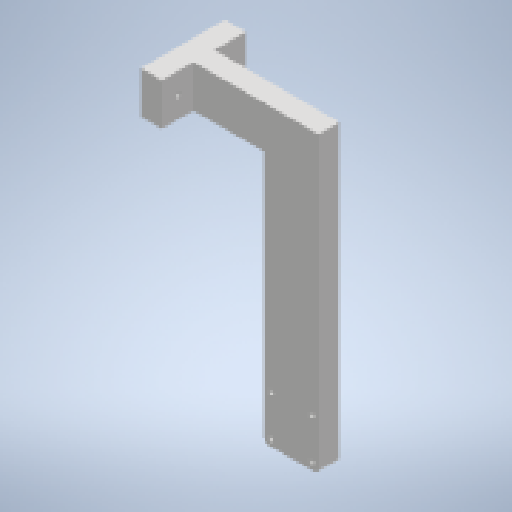
# Autodesk Inventor part: patas2
Saved by Autodesk Inventor 2023.2 (Build 272271030, 271C)
## iProperties
Created: 2023-03-05
Part Number: patas2
Material: Generic
Document SubType Name: Sheet Metal
Designer: angel
Density: 1 g/cm^3
Sheet Metal Rule: Default_mm
Appearance: Default
Author: angel
Autodesk Inventor part; units mm, degrees
ref_plane "YZ Plane" through (0, 0, 0) normal (1, 0, 0) x (0, 1, 0)
ref_plane "XZ Plane" through (0, 0, 0) normal (0, 1, 0) x (-1, 0, 0)
ref_plane "XY Plane" through (0, 0, 0) normal (0, 0, 1) x (1, 0, 0)
sketch "Sketch1" plane through (0, 0, 0) normal (0, 0, 1) x (1, 0, 0)
  line L0 (11.35, 40) -> (11.35, -15)
  line L1 (6.35, -20) -> (-48.65, -20)
  circle A0 centre (2.814466, -11.464466) radius 3
  circle A1 centre (-45.114466, -11.464466) radius 3
  circle A2 centre (-45.114466, 36.464466) radius 3
  circle A3 centre (2.814466, 36.464466) radius 3
  line L2 (-162.568945, -644.9995) -> (-162.568945, 135.0005)
  line L3 (11.35, -15) -> (11.35, 330)
  line L4 (-53.65, -15) -> (-53.65, 40)
  line L5 (-53.65, -15) -> (-53.65, 280)
  line L6 (11.35, 330) -> (-162.568945, 330)
  line L7 (-162.568945, 330) -> (-162.568945, 280)
  line L8 (-162.568945, 280) -> (-53.65, 280)
  line L9 (6.35, -20) -> (-48.65, -20)
  arc A4 (6.35, -20) -> (11.35, -15) centre (6.35, -15) ccw
  arc A5 (-53.65, -15) -> (-48.65, -20) centre (-48.65, -15) ccw
  circle A6 centre (2.814466, 36.464466) radius 3
  circle A7 centre (2.814466, -11.464466) radius 3
  circle A8 centre (-45.114466, -11.464466) radius 3
  circle A9 centre (-45.114466, 36.464466) radius 3
  point P0 (0, 0)
  dimension "d0" = 350
  dimension "d1" = 300
  dimension "d2" = 5
  measures "d0" distance from line of L3.end L1
  measures "d1" distance from line of L5.end L1
  measures "d2" radius of A4
sketch "Sketch2" plane through (-162.568945, 280, 0) normal (-1, 0, 0) x (0, 0, 1)
  line L0 (0, 0) -> (25, 0)
  line L1 (0, 50) -> (25, 50)
  line L2 (25, 0) -> (25, 50)
  line L3 (-37.5, 50) -> (62.5, 50)
  line L4 (62.5, 50) -> (62.5, 0)
  line L5 (62.5, 0) -> (-37.5, 0)
  line L6 (-37.5, 0) -> (-37.5, 50)
  circle A0 centre (42.5, 25) radius 3
  circle A1 centre (-17.5, 25) radius 3
  point P0 (0, -280)
  point P1 (12.5, 50)
  point P2 (12.5, 50)
  point P3 (62.5, 25)
  point P4 (-37.5, 25)
  dimension "d4" = 50
  dimension "d5" = 50
  dimension "d6" = 25
  dimension "d7" = 20
  dimension "d8" = 20
  dimension "d9" = 6
  measures "d4" distance from line of L4 point (12.5, 50)
  measures "d5" distance from line of L6 point (12.5, 50)
  measures "d6" distance from line of L3 point (62.5, 25)
  measures "d7" distance of A1.centre point (-37.5, 25)
  measures "d8" distance from line of L4 A0.centre
  measures "d9" diameter of A0
sketch "Sketch1 outline for Plate1" plane through (0, 0, 0) normal (0, 0, 1) x (1, 0, 0)
  arc A0 (6.35, -20) -> (11.35, -15) centre (6.35, -15) ccw
  line L0 (-48.65, -20) -> (6.35, -20)
  line L1 (11.35, -15) -> (11.35, 330)
  arc A1 (-53.65, -15) -> (-48.65, -20) centre (-48.65, -15) ccw
  line L2 (11.35, 330) -> (-162.568945, 330)
  line L3 (-53.65, 280) -> (-53.65, -15)
  line L4 (-162.568945, 330) -> (-162.568945, 280)
  line L5 (-162.568945, 280) -> (-53.65, 280)
  circle A2 centre (-45.114466, -11.464466) radius 3
  circle A3 centre (2.814466, -11.464466) radius 3
  circle A4 centre (-45.114466, 36.464466) radius 3
  circle A5 centre (2.814466, 36.464466) radius 3
extrude "Plate1" add sketch "Sketch1 outline for Plate1" along normal blind 25
sketch "Sketch2 outline for Plate2" plane through (-162.568945, 280, 0) normal (-1, 0, 0) x (0, 0, 1)
  line L0 (-37.5, 50) -> (62.5, 50)
  line L1 (-37.5, 0) -> (-37.5, 50)
  line L2 (62.5, 50) -> (62.5, 0)
  line L3 (62.5, 0) -> (-37.5, 0)
  circle A0 centre (-17.5, 25) radius 3
  circle A1 centre (42.5, 25) radius 3
sheet face with bend "Face2" sketch "Sketch2 outline for Plate2" thickness 25 toward (1, 0, 0) bend radius 25
bend "Bend1"
equation "\"d3\" = Thickness"
equation "\"d10\" = BendRadius"
equation "\"d11\" = BendReliefWidth"
equation "\"d13\" = MinimumRemnant"
equation "\"d12\" = BendReliefDepth"
equation "\"d14\" = TransitionRadius"
equation "\"BendRadius\" = Thickness"
equation "\"BendReliefWidth\" = Thickness"
equation "\"BendReliefDepth\" = 0.5 * Thickness"
equation "\"TransitionRadius\" = BendRadius"
equation "\"JacobiRadiusSize\" = BendRadius"
equation "\"GapSize\" = Thickness"
equation "\"Thickness\" = 25"
equation "\"MinimumRemnant\" = 50"
body "Solid1"
